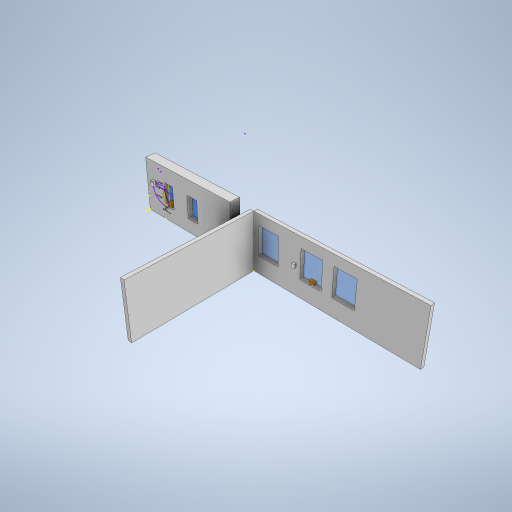
# Autodesk Inventor part: Scene
Saved by Autodesk Inventor 2024 (Build 280153000, 153)
## iProperties
Created: 2023-09-14
Part Number: Scene
Material: Generic
Document SubType Name: Modeling
Designer: vegaj
Density: 1 g/cm^3
Appearance: Default
Author: vegaj
Autodesk Inventor part; units mm, degrees
ref_plane "YZ Plane" through (0, 0, 0) normal (1, 0, 0) x (0, 1, 0)
ref_plane "XZ Plane" through (0, 0, 0) normal (0, 1, 0) x (-1, 0, 0)
ref_plane "XY Plane" through (0, 0, 0) normal (0, 0, 1) x (1, 0, 0)
sketch "Sketch5" plane through (0, 0, 0) normal (0, 0, 1) x (1, 0, 0)
  line L0 (0, 0) -> (508, 0)
  line L1 (508, 0) -> (508, 254)
  line L2 (508, 254) -> (0, 254)
  line L3 (0, 254) -> (0, 0)
  line L4 (106.3948, 178.5315) -> (165.5889, 178.5315)
  line L5 (165.5889, 178.5315) -> (165.5889, 68.5809)
  line L6 (165.5889, 68.5809) -> (106.3948, 68.5809)
  line L7 (106.3948, 68.5809) -> (106.3948, 178.5315)
  line L8 (254.8332, 177.8) -> (314.0855, 177.8)
  line L9 (314.0855, 177.8) -> (314.0855, 67.8493)
  line L10 (314.0855, 67.8493) -> (254.8332, 67.8493)
  line L11 (254.8332, 67.8493) -> (254.8332, 177.8)
  dimension "d14" = 508
  dimension "d15" = 254
  constraints: 24 end point, 6 parallel, 3 horizontal, 3 perpendicular
  measures "d14" distance of L2.end L1.end
  measures "d15" distance of L1.end L0.end
extrude "Extrusion4" add sketch "Sketch5" against normal blind 50.8
sketch "Sketch8" plane through (106.3948, 68.5809, 0) normal (0, 1, 0) x (1, 0, 0)
  line L0 (0, 0) -> (0, 50.8) projected
  line L1 (0, 25.4) -> (59.1942, 25.4)
  line L2 (59.1942, 25.4) -> (59.1942, 50.8)
  line L3 (59.1942, 50.8) -> (0, 50.8)
  line L4 (0, 50.8) -> (0, 25.4)
  point P0 (-106.3948, 0)
  constraints: 8 end point, 2 parallel, 1 horizontal, 1 midpoint, 1 perpendicular
extrude "Extrusion6" add sketch "Sketch8" along normal blind 107.95
sketch "Sketch9" plane through (254.8332, 67.8493, 0) normal (0, 1, 0) x (1, 0, 0)
  line L0 (0, 0) -> (0, 50.8) projected
  line L1 (0, 25.4) -> (59.2523, 25.4)
  line L2 (59.2523, 25.4) -> (59.2523, 50.8)
  line L3 (59.2523, 50.8) -> (0, 50.8)
  line L4 (0, 50.8) -> (0, 25.4)
  point P0 (-254.8332, 0)
  constraints: 8 end point, 2 parallel, 1 horizontal, 1 midpoint, 1 perpendicular
extrude "Extrusion7" add sketch "Sketch9" along normal blind 107.95
sketch "Sketch10" plane through (106.3948, 68.5809, 0) normal (0, 1, 0) x (1, 0, 0)
  line L0 (16.891, 25.4) -> (42.291, 25.4)
  line L1 (42.291, 25.4) -> (42.291, 5.08)
  line L2 (42.291, 5.08) -> (16.891, 5.08)
  line L3 (16.891, 5.08) -> (16.891, 25.4)
  point P0 (-106.3948, 0)
  dimension "d35" = 25.4
  dimension "d36" = 20.32
  constraints: 8 end point, 2 parallel, 1 horizontal, 1 perpendicular
  measures "d35" distance of L1.end L2.end
  measures "d36" distance of L0.end L1.end
extrude "Extrusion8" add sketch "Sketch10" along normal blind 17.4625
sketch "Sketch11" plane through (106.3948, 176.5309, -25.4) normal (0, 0, 1) x (1, 0, 0)
  circle A0 centre (29.591, -63.8397) radius 3.81
  point P0 (-106.3948, -176.5309)
  dimension "d40" = 7.62
  constraints: 1 centre point
  measures "d40" diameter of A0
extrude "Extrusion9" add sketch "Sketch11" along normal blind 9.525
sketch "Sketch12" plane through (106.3948, 68.5809, 0) normal (0, 1, 0) x (1, 0, 0)
  line L0 (42.291, 5.08) -> (16.891, 5.08) projected
  line L1 (27.94, 5.08) -> (30.607, 5.08)
  line L2 (30.607, 5.08) -> (30.607, -20.32)
  line L3 (30.607, -20.32) -> (27.94, -20.32)
  line L4 (27.94, -20.32) -> (27.94, 5.08)
  point P0 (-106.3948, 0)
  dimension "d43" = 2.667
  dimension "d44" = 25.4
  constraints: 8 end point, 2 parallel, 1 horizontal, 1 perpendicular, 1 point on line
  measures "d43" distance of L2.end L3.end
  measures "d44" distance of L1.end L2.end
extrude "Extrusion10" add sketch "Sketch12" along normal blind 4.445
sketch "Sketch13" plane through (134.3348, 68.5809, 20.32) normal (0, 0, 1) x (1, 0, 0)
  circle A0 centre (1.3335, 8.255) radius 3.81
  point P0 (-134.3348, -68.5809)
  dimension "d47" = 7.62
  constraints: 1 centre point
  measures "d47" diameter of A0
extrude "Extrusion11" add sketch "Sketch13" against normal blind 4.445
sketch "Sketch16" plane through (106.3948, 176.5309, -25.4) normal (0, 0, 1) x (1, 0, 0)
  line L0 (14.3059, -54.6716) -> (46.9521, -54.6716) construction
  line L1 (46.9521, -54.6716) -> (46.9521, -58.6978) construction
  line L2 (46.9521, -58.6978) -> (14.3059, -58.6978) construction
  line L3 (14.3059, -58.6978) -> (14.3059, -54.6716) construction
  point P0 (-106.3948, -176.5309)
  constraints: 2 other
sketch "Sketch17" plane through (106.3948, 176.5309, -25.4) normal (0, 0, 1) x (1, 0, 0)
  line L0 (15.7059, -85.8021) -> (44.6397, -85.8021) construction
  line L1 (44.6397, -85.8021) -> (44.6397, -89.8282) construction
  line L2 (44.6397, -89.8282) -> (15.7059, -89.8282) construction
  line L3 (15.7059, -89.8282) -> (15.7059, -85.8021) construction
  point P0 (-106.3948, -176.5309)
  constraints: 2 other
sketch "Sketch18" plane through (135.6683, 76.8359, 20.32) normal (0, 0, 1) x (1, 0, 0)
  line L0 (-19.3162, -9.5529) -> (36.6939, -9.5529) construction
  line L1 (36.6939, -9.5529) -> (36.6939, -13.579) construction
  line L2 (36.6939, -13.579) -> (-19.3162, -13.579) construction
  line L3 (-19.3162, -13.579) -> (-19.3162, -9.5529) construction
  point P0 (-135.6683, -76.8359)
  constraints: 2 other
sketch "Sketch19" plane through (0, 0, 0) normal (0, 0, 1) x (1, 0, 0)
  line L0 (106.3948, 68.5809) -> (106.3948, 176.5309) projected
  arc A0 (56.654, 159.4739) -> (106.3948, 159.8999) centre (80.9132, 231.0621) ccw
  point P0 (0, 0)
  constraints: 2 point on circle, 1 centre point, 1 point on line
sketch "Sketch21" plane through (106.3948, 68.5809, 0) normal (1, 0, 0) x (0, 0, -1)
  line L0 (0, 0) -> (0, 109.9507) projected
  line L1 (25.4, 0) -> (25.4, 107.95) projected
  arc A0 (0, 91.1415) -> (25.4, 43.4398) centre (113.4917, 120.9598) ccw
  point P0 (0, -68.5809)
  constraints: 2 point on circle, 2 point on line, 1 centre point
sketch "Sketch22" plane through (106.3948, 176.5309, -25.4) normal (0, 0, 1) x (1, 0, 0)
  line L0 (0, -107.95) -> (0, 0) projected
  circle A0 centre (29.591, -63.8397) radius 3.81 projected
  arc A1 (0, -65.62) -> (25.781, -63.8397) centre (10.1339, -24.8109) ccw
  point P0 (-106.3948, -176.5309)
  constraints: 2 point on circle, 1 centre point, 1 horizontal alignment, 1 point on line, 1 other
sketch "Sketch24" plane through (0, 0, 0) normal (0, 0, 1) x (1, 0, 0)
  line L0 (63.5, 165.1) -> (63.5, 127) projected
  arc A0 (63.5, 150.7683) -> (106.3948, 144.9276) centre (98.4452, 246.9769) ccw
  point P0 (0, 0)
  constraints: 2 point on circle, 1 centre point, 1 point on line
sketch "Sketch25" plane through (106.3948, 68.5809, 0) normal (1, 0, 0) x (0, 0, -1)
  line L0 (0, 0) -> (25.4, 0) projected
  arc A0 (0, 75.9575) -> (20.5025, 0) centre (471.8024, 162.5611) ccw
  point P0 (0, -68.5809)
  constraints: 2 point on circle, 1 centre point, 1 point on line
sketch "Sketch26" plane through (106.3948, 68.5809, 0) normal (0, 1, 0) x (1, 0, 0)
  line L0 (0, 0) -> (0, 25.4) projected
  line L1 (16.891, 5.08) -> (16.891, 25.4) projected
  arc A0 (0, 20.7585) -> (16.891, 14.7493) centre (10.6546, 23.9633) ccw
  point P0 (-106.3948, 0)
  constraints: 2 point on circle, 2 point on line, 1 centre point
sketch "Sketch28" plane through (0, 0, 0) normal (0, 0, 1) x (1, 0, 0)
  line L0 (134.3348, 68.5809) -> (106.3948, 68.5809) projected
  line L1 (137.0018, 68.5809) -> (134.3348, 68.5809) projected
  arc A0 (131.2385, 68.5809) -> (134.3348, 68.5809) centre (132.7866, 73.5411) ccw
  arc A1 (35.3873, 159.2878) -> (131.2385, 65.871) centre (111.28, 141.2753) ccw
  line L2 (106.3948, 68.5809) -> (106.3948, 178.5315) projected
  arc A2 (56.8389, 152.8761) -> (106.3948, 144.0937) centre (94.7313, 222.4849) ccw
  point P0 (0, 0)
  constraints: 6 point on circle, 3 centre point, 2 point on line
sketch "Sketch30" plane through (0, 0, 0) normal (0, 0, 1) x (1, 0, 0)
  line L0 (64.7632, 170.4894) -> (105.7037, 170.4894) construction
  line L1 (105.7037, 170.4894) -> (105.7037, 161.4449) construction
  line L2 (105.7037, 161.4449) -> (64.7632, 161.4449) construction
  line L3 (64.7632, 161.4449) -> (64.7632, 170.4894) construction
  line L4 (60.3339, 142.2504) -> (104.8125, 142.2504) construction
  line L5 (104.8125, 142.2504) -> (104.8125, 133.2058) construction
  line L6 (104.8125, 133.2058) -> (60.3339, 133.2058) construction
  line L7 (60.3339, 133.2058) -> (60.3339, 142.2504) construction
  line L8 (53.7063, 100.1518) -> (93.849, 100.1518) construction
  line L9 (93.849, 100.1518) -> (93.849, 90.0633) construction
  line L10 (93.849, 90.0633) -> (53.7063, 90.0633) construction
  line L11 (53.7063, 90.0633) -> (53.7063, 100.1518) construction
  point P0 (0, 0)
  constraints: 6 other
sketch "Sketch32" plane through (0, 0, 0) normal (0, 0, 1) x (1, 0, 0)
  line L0 (57.2103, 163.3925) -> (37.4567, 163.3925)
  line L1 (37.4567, 163.3925) -> (37.4567, 137.9925)
  line L2 (37.4567, 137.9925) -> (57.2103, 137.9925)
  line L3 (57.2103, 137.9925) -> (57.2103, 163.3925)
  point P0 (0, 0)
  dimension "d51" = 19.7536
  dimension "d52" = 25.4
  constraints: 8 end point, 2 parallel, 1 horizontal, 1 perpendicular
  measures "d51" distance of L2.end L1.end
  measures "d52" distance of L1.end L0.end
extrude "Extrusion12" add sketch "Sketch32" along normal blind 12.7
sketch "Sketch33" plane through (0, 0, 12.7) normal (0, 0, 1) x (1, 0, 0)
  line L0 (37.7328, 161.9101) -> (67.7929, 161.9101) construction
  line L1 (67.7929, 161.9101) -> (67.7929, 152.5818) construction
  line L2 (67.7929, 152.5818) -> (37.7328, 152.5818) construction
  line L3 (37.7328, 152.5818) -> (37.7328, 161.9101) construction
  point P0 (0, 0)
  constraints: 2 other
sketch "Sketch34" plane through (57.2103, 137.9925, 0) normal (1, 0, 0) x (0, 0, -1)
  point P0 (0, -137.9925)
  point P1 (-2.5352, 21.6579)
  point P2 (-2.6184, 15.5355)
  point P3 (-2.7643, 9.6031)
  point P4 (-2.9557, 3.2698)
hole "Hole2" at (57.2103, 159.6504, 2.5352) at (57.2103, 153.528, 2.6184) at (57.2103, 141.2623, 2.9557) at (57.2103, 147.5956, 2.7643) direction (-1, 0, 0) diameter 3.175 depth 131.445 tip angle 126
sketch "Sketch35" plane through (0, 0, 0) normal (0, -1, 0) x (1, 0, 0)
  point P0 (0, 0)
sketch "Sketch36" plane through (0, 0, 0) normal (0, 0, 1) x (1, 0, 0)
  line L0 (635, 0) -> (1413.764, 0)
  line L1 (1413.764, 0) -> (1413.764, 270.764)
  line L2 (1413.764, 270.764) -> (635, 270.764)
  line L3 (635, 270.764) -> (635, 0)
  line L4 (871.982, 84.582) -> (973.582, 84.582)
  line L5 (973.582, 84.582) -> (973.582, 219.964)
  line L6 (973.582, 219.964) -> (871.982, 219.964)
  line L7 (871.982, 219.964) -> (871.982, 84.582)
  line L8 (1024.382, 84.582) -> (1125.982, 84.582)
  line L9 (1125.982, 84.582) -> (1125.982, 219.964)
  line L10 (1125.982, 219.964) -> (1024.382, 219.964)
  line L11 (1024.382, 219.964) -> (1024.382, 84.582)
  line L12 (660.4, 84.582) -> (762, 84.582)
  line L13 (762, 84.582) -> (762, 219.964)
  line L14 (762, 219.964) -> (660.4, 219.964)
  line L15 (660.4, 219.964) -> (660.4, 84.582)
  point P0 (0, 0)
  dimension "d62" = 778.764
  dimension "d63" = 270.764
  dimension "d64" = 101.6
  dimension "d65" = 135.382
  dimension "d66" = 101.6
  dimension "d67" = 135.382
  dimension "d68" = 101.6
  dimension "d69" = 135.382
  constraints: 32 end point, 8 parallel, 4 horizontal, 4 perpendicular, 2 point on line
  measures "d62" distance of L2.end L1.end
  measures "d63" distance of L1.end L0.end
  measures "d64" distance of L6.end L5.end
  measures "d65" distance of L5.end L4.end
  measures "d66" distance of L10.end L9.end
  measures "d67" distance of L9.end L8.end
  measures "d68" distance of L14.end L13.end
  measures "d69" distance of L13.end L12.end
extrude "Extrusion13" add sketch "Sketch36" against normal blind 19.05
sketch "Sketch37" plane through (635, 0, 0) normal (-1, 0, 0) x (0, 0, 1)
  point P0 (0, 0)
sketch "Sketch38" plane through (635, 0, 0) normal (-1, 0, 0) x (0, 0, 1)
  line L0 (0, 0) -> (-19.05, 0) projected
  line L1 (0, 0) -> (592.582, 0)
  line L2 (592.582, 0) -> (592.582, 270.764)
  line L3 (592.582, 270.764) -> (0, 270.764)
  line L4 (0, 270.764) -> (0, 0)
  dimension "d72" = 592.582
  dimension "d73" = 270.764
  constraints: 8 end point, 2 parallel, 1 horizontal, 1 perpendicular
  measures "d72" distance of L3.end L2.end
  measures "d73" distance of L2.end L1.end
extrude "Extrusion14" add sketch "Sketch38" along normal blind 19.05
sketch "Sketch39" plane through (871.982, 84.582, 0) normal (0, 1, 0) x (1, 0, 0)
  line L0 (0, 19.05) -> (101.6, 19.05) projected
  line L1 (0, 19.05) -> (101.6, 19.05)
  line L2 (101.6, 19.05) -> (101.6, 31.75)
  line L3 (101.6, 31.75) -> (0, 31.75)
  line L4 (0, 31.75) -> (0, 19.05)
  line L5 (152.4, 19.05) -> (254, 19.05)
  line L6 (254, 19.05) -> (254, 31.75)
  line L7 (254, 31.75) -> (152.4, 31.75)
  line L8 (152.4, 31.75) -> (152.4, 19.05)
  line L9 (-211.582, 0) -> (-211.582, 19.05) projected
  line L10 (-211.582, 19.05) -> (-109.982, 19.05)
  line L11 (-109.982, 19.05) -> (-109.982, 31.75)
  line L12 (-109.982, 31.75) -> (-211.582, 31.75)
  line L13 (-211.582, 31.75) -> (-211.582, 19.05)
  point P0 (-871.982, 0)
  dimension "d76" = 101.6
  dimension "d77" = 12.7
  dimension "d78" = 101.6
  dimension "d79" = 12.7
  dimension "d80" = 101.6
  dimension "d81" = 12.7
  constraints: 24 end point, 6 parallel, 3 horizontal, 3 perpendicular
  measures "d76" distance of L3.end L2.end
  measures "d77" distance of L2.end L1.end
  measures "d78" distance of L7.end L6.end
  measures "d79" distance of L6.end L5.end
  measures "d80" distance of L12.end L11.end
  measures "d81" distance of L11.end L10.end
extrude "Extrusion15" add sketch "Sketch39" along normal blind 135.382
sketch "Sketch40" plane through (0, 0, 0) normal (0, 0, 1) x (1, 0, 0)
  line L0 (838.2, 127) -> (850.9, 127)
  line L1 (850.9, 127) -> (850.9, 143.9164)
  line L2 (850.9, 143.9164) -> (838.2, 143.9164)
  line L3 (838.2, 143.9164) -> (838.2, 127)
  point P0 (0, 0)
  dimension "d84" = 12.7
  dimension "d85" = 16.9164
  constraints: 8 end point, 2 parallel, 1 horizontal, 1 perpendicular
  measures "d84" distance of L2.end L1.end
  measures "d85" distance of L1.end L0.end
extrude "Extrusion16" add sketch "Sketch40" along normal blind 10.5816
sketch "Sketch41" plane through (850.9, 127, 0) normal (1, 0, 0) x (0, 0, -1)
  point P0 (0, -127)
  point P1 (-2.1386, 14.5927)
  point P2 (-2.1394, 10.841)
  point P3 (-2.207, 6.7203)
  point P4 (-2.2926, 2.8121)
hole "Hole3" at (850.9, 137.841, 2.1394) at (850.9, 141.5927, 2.1386) at (850.9, 133.7203, 2.207) at (850.9, 129.8121, 2.2926) direction (-1, 0, 0) diameter 2.54 depth 190.5
sketch "Sketch42" plane through (871.982, 84.582, -19.05) normal (0, 0, 1) x (1, 0, 0)
  circle A0 centre (50.8, 50.8) radius 0.4064
  point P0 (-871.982, -84.582)
  dimension "d95" = 0.8128
  constraints: 1 centre point
  measures "d95" diameter of A0
extrude "Extrusion17" add sketch "Sketch42" along normal blind 0.508
sketch "Sketch46" plane through (871.982, 84.582, -19.05) normal (0, 0, 1) x (1, 0, 0)
  line L0 (38.1, 0) -> (63.5, 0)
  line L1 (63.5, 0) -> (63.5, 12.7)
  line L2 (63.5, 12.7) -> (38.1, 12.7)
  line L3 (38.1, 12.7) -> (38.1, 0)
  point P0 (-871.982, -84.582)
  dimension "d98" = 25.4
  dimension "d99" = 12.7
  constraints: 8 end point, 2 parallel, 1 horizontal, 1 perpendicular
  measures "d98" distance of L2.end L1.end
  measures "d99" distance of L1.end L0.end
extrude "Extrusion18" add sketch "Sketch46" along normal blind 12.7
sketch "Sketch47" plane through (871.982, 84.582, 0) normal (0, 1, 0) x (1, 0, 0)
  line L0 (63.5, 6.35) -> (38.1, 6.35) projected
  line L1 (48.26, 6.35) -> (49.8998, 6.35)
  line L2 (49.8998, 6.35) -> (49.8998, -4.2164)
  line L3 (49.8998, -4.2164) -> (48.26, -4.2164)
  line L4 (48.26, -4.2164) -> (48.26, 6.35)
  point P0 (-871.982, 0)
  dimension "d102" = 10.5664
  constraints: 8 end point, 2 parallel, 1 horizontal, 1 perpendicular, 1 point on line
  measures "d102" distance of L1.end L2.end
extrude "Extrusion19" add sketch "Sketch47" along normal blind 0.635
sketch "Sketch48" plane through (920.242, 84.582, 4.2164) normal (0, 0, 1) x (1, 0, 0)
  circle A0 centre (0.8199, 1.0414) radius 0.4064
  point P0 (-920.242, -84.582)
  constraints: 1 centre point
extrude "Extrusion20" add sketch "Sketch48" against normal blind 0.3556
body "Solid5"
